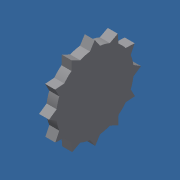
# Autodesk Inventor part: CarotGear
Saved by Autodesk Inventor 2018 (Build 220112000, 112)
## iProperties
Created: 2022-02-21
Part Number: CarotGear
Material: Generic
Document SubType Name: Modeling
Designer: Nathann
Density: 1 g/cm^3
Appearance: Default
Author: Nathann
Autodesk Inventor part; units mm, degrees
ref_plane "YZ Plane" through (0, 0, 0) normal (1, 0, 0) x (0, 1, 0)
ref_plane "XZ Plane" through (0, 0, 0) normal (0, 1, 0) x (-1, 0, 0)
ref_plane "XY Plane" through (0, 0, 0) normal (0, 0, 1) x (1, 0, 0)
sketch "Sketch1" plane through (0, 0, 0) normal (1, 0, 0) x (0, 1, 0)
  line L0 (22.9447, 2.9962) -> (27.4904, 0.1436)
  line L1 (27.4904, 0.1436) -> (22.9447, -2.9962)
  line L2 (18.3726, 14.0671) -> (23.7356, 13.8695)
  line L3 (23.7356, 13.8695) -> (21.3688, 8.8776)
  line L4 (8.8776, 21.3688) -> (13.6209, 23.8791)
  line L5 (13.6209, 23.8791) -> (14.0671, 18.3726)
  line L6 (-2.9962, 22.9447) -> (-0.1436, 27.4904)
  line L7 (-0.1436, 27.4904) -> (2.9962, 22.9447)
  line L8 (-14.0671, 18.3726) -> (-13.8695, 23.7356)
  line L9 (-13.8695, 23.7356) -> (-8.8776, 21.3688)
  line L10 (-21.3688, 8.8776) -> (-23.8791, 13.6209)
  line L11 (-23.8791, 13.6209) -> (-18.3726, 14.0671)
  line L12 (-22.9447, -2.9962) -> (-27.4904, -0.1436)
  line L13 (-27.4904, -0.1436) -> (-22.9447, 2.9962)
  line L14 (-18.3726, -14.0671) -> (-23.7356, -13.8695)
  line L15 (-23.7356, -13.8695) -> (-21.3688, -8.8776)
  line L16 (-8.8776, -21.3688) -> (-13.6209, -23.8791)
  line L17 (-13.6209, -23.8791) -> (-14.0671, -18.3726)
  line L18 (2.9962, -22.9447) -> (0.1436, -27.4904)
  line L19 (0.1436, -27.4904) -> (-2.9962, -22.9447)
  line L20 (14.0671, -18.3726) -> (13.8695, -23.7356)
  line L21 (13.8695, -23.7356) -> (8.8776, -21.3688)
  line L22 (21.3688, -8.8776) -> (23.8791, -13.6209)
  line L23 (23.8791, -13.6209) -> (18.3726, -14.0671)
  arc A0 (22.9447, 2.9962) -> (21.3688, 8.8776) centre (0, 0) ccw
  arc A1 (18.3726, 14.0671) -> (14.0671, 18.3726) centre (0, 0) ccw
  arc A2 (8.8776, 21.3688) -> (2.9962, 22.9447) centre (0, 0) ccw
  arc A3 (-2.9962, 22.9447) -> (-8.8776, 21.3688) centre (0, 0) ccw
  arc A4 (-14.0671, 18.3726) -> (-18.3726, 14.0671) centre (0, 0) ccw
  arc A5 (-21.3688, 8.8776) -> (-22.9447, 2.9962) centre (0, 0) ccw
  arc A6 (-22.9447, -2.9962) -> (-21.3688, -8.8776) centre (0, 0) ccw
  arc A7 (-18.3726, -14.0671) -> (-14.0671, -18.3726) centre (0, 0) ccw
  arc A8 (-8.8776, -21.3688) -> (-2.9962, -22.9447) centre (0, 0) ccw
  arc A9 (2.9962, -22.9447) -> (8.8776, -21.3688) centre (0, 0) ccw
  arc A10 (14.0671, -18.3726) -> (18.3726, -14.0671) centre (0, 0) ccw
  arc A11 (21.3688, -8.8776) -> (22.9447, -2.9962) centre (0, 0) ccw
  dimension "d2" = 360
  constraints: 48 end point, 24 point on circle, 12 centre point, 1 coincident, 61 other
extrude "Extrusion1" add sketch "Sketch1" along normal blind 6
body "Solid1"
